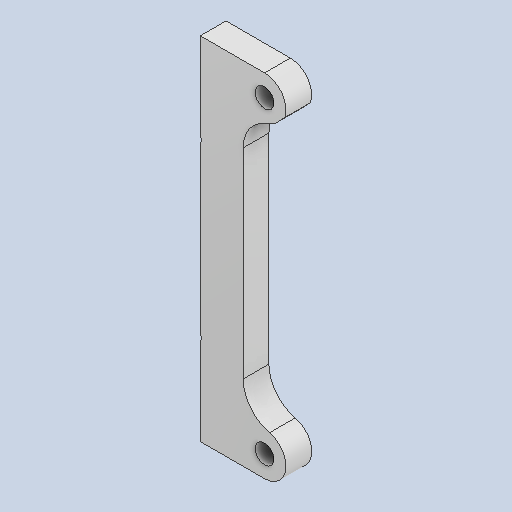
# Autodesk Inventor part: asikubi_asi
Saved by Autodesk Inventor 2025.1 (Build 291241000, 241)
## iProperties
Created: 2024-09-04
Part Number: asikubi_asi
Material: アルミニウム 2014-T4
Document SubType Name: Modeling
Designer: right
Mass: 2.02961 g
Surface Area: 8.92345 cm^2
Volume: 0.724859 cm^3
Density: 2.8 g/cm^3
Appearance: サテン
Author: right
Autodesk Inventor part; units mm, degrees
note: some values were not read from the file. Chosen so that the rebuilt part matches the saved one: edges of "フィレット3".
ref_plane "YZ Plane" through (0, 0, 0) normal (1, 0, 0) x (0, 1, 0)
ref_plane "XZ Plane" through (0, 0, 0) normal (0, 1, 0) x (-1, 0, 0)
ref_plane "XY Plane" through (0, 0, 0) normal (0, 0, 1) x (1, 0, 0)
sketch "スケッチ1" plane through (0, 0, 0) normal (0, 0, 1) x (1, 0, 0)
  line L0 (22.7151, -43.926) -> (22.7151, -4.926) construction
  arc A0 (22.2151, -44.426) -> (22.7151, -43.926) centre (22.2151, -43.926) ccw construction
  line L1 (3.2151, -44.426) -> (22.2151, -44.426) construction
  arc A1 (2.7151, -43.926) -> (3.2151, -44.426) centre (3.2151, -43.926) ccw construction
  line L2 (2.7151, -4.926) -> (2.7151, -43.926) construction
  arc A2 (3.2151, -4.426) -> (2.7151, -4.926) centre (3.2151, -4.926) ccw construction
  line L3 (22.2151, -4.426) -> (3.2151, -4.426) construction
  arc A3 (22.7151, -4.926) -> (22.2151, -4.426) centre (22.2151, -4.926) ccw construction
  line L4 (6.2865, -24.2474) -> (6.2865, -30.6046) construction
  line L5 (6.2865, -30.6046) -> (10.1437, -30.6046) construction
  line L6 (10.1437, -30.6046) -> (10.1437, -24.2474) construction
  line L7 (10.1437, -24.2474) -> (6.2865, -24.2474) construction
  circle A4 centre (12.7151, -31.826) radius 1.1519 construction
  line L8 (19.1437, -24.2474) -> (15.2865, -24.2474) construction
  line L9 (15.2865, -24.2474) -> (15.2865, -30.6046) construction
  line L10 (15.2865, -30.6046) -> (19.1437, -30.6046) construction
  line L11 (19.1437, -30.6046) -> (19.1437, -24.2474) construction
  circle A5 centre (4.7151, -6.426) radius 1.8131 construction
  circle A6 centre (20.7151, -6.426) radius 1.8131 construction
  circle A7 centre (4.7151, -42.426) radius 1.8131 construction
  circle A8 centre (20.7151, -42.426) radius 1.8131 construction
  arc A9 (18.9651, -12.926) -> (6.4651, -12.9153) centre (12.7151, -12.926) ccw construction
  arc A10 (6.4649, -12.9153) -> (6.2151, -12.676) centre (6.2151, -12.926) ccw construction
  line L12 (6.2151, -12.676) -> (4.4651, -12.676) construction
  arc A11 (4.4651, -12.676) -> (4.4651, -13.176) centre (4.4651, -12.926) ccw construction
  line L13 (4.4651, -13.176) -> (6.2151, -13.176) construction
  arc A12 (6.2151, -13.176) -> (6.4651, -12.926) centre (6.2151, -12.926) ccw construction
  arc A13 (6.4651, -12.926) -> (6.9408, -15.3178) centre (12.7151, -12.926) ccw construction
  arc A14 (6.9408, -15.3178) -> (6.6142, -15.1825) centre (6.7099, -15.4134) ccw construction
  line L14 (6.6142, -15.1825) -> (4.9974, -15.8522) construction
  arc A15 (4.9974, -15.8522) -> (5.1888, -16.3141) centre (5.0931, -16.0831) ccw construction
  line L15 (5.1888, -16.3141) -> (6.8055, -15.6444) construction
  arc A16 (6.8055, -15.6444) -> (6.9408, -15.3178) centre (6.7099, -15.4134) ccw construction
  arc A17 (6.9408, -15.3178) -> (8.2957, -17.3454) centre (12.7151, -12.926) ccw construction
  arc A18 (8.2957, -17.3454) -> (7.9421, -17.3454) centre (8.1189, -17.5222) ccw construction
  line L16 (7.9421, -17.3454) -> (6.7047, -18.5829) construction
  arc A19 (6.7047, -18.5829) -> (7.0582, -18.9364) centre (6.8815, -18.7596) ccw construction
  line L17 (7.0582, -18.9364) -> (8.2957, -17.699) construction
  arc A20 (8.2957, -17.699) -> (8.2957, -17.3454) centre (8.1189, -17.5222) ccw construction
  arc A21 (8.2957, -17.3454) -> (10.3233, -18.7003) centre (12.7151, -12.926) ccw construction
  arc A22 (10.3233, -18.7003) -> (9.9967, -18.8356) centre (10.2277, -18.9312) ccw construction
  line L18 (9.9967, -18.8356) -> (9.327, -20.4523) construction
  arc A23 (9.327, -20.4523) -> (9.7889, -20.6437) centre (9.558, -20.548) ccw construction
  line L19 (9.7889, -20.6437) -> (10.4586, -19.0269) construction
  arc A24 (10.4586, -19.0269) -> (10.3233, -18.7003) centre (10.2277, -18.9312) ccw construction
  arc A25 (10.3233, -18.7003) -> (12.7151, -19.176) centre (12.7151, -12.926) ccw construction
  arc A26 (12.7151, -19.176) -> (12.4651, -19.426) centre (12.7151, -19.426) ccw construction
  line L20 (12.4651, -19.426) -> (12.4651, -21.176) construction
  arc A27 (12.4651, -21.176) -> (12.9651, -21.176) centre (12.7151, -21.176) ccw construction
  line L21 (12.9651, -21.176) -> (12.9651, -19.426) construction
  arc A28 (12.9651, -19.426) -> (12.7151, -19.176) centre (12.7151, -19.426) ccw construction
  arc A29 (12.7151, -19.176) -> (15.1069, -18.7003) centre (12.7151, -12.926) ccw construction
  arc A30 (15.1069, -18.7003) -> (14.9716, -19.0269) centre (15.2025, -18.9312) ccw construction
  line L22 (14.9716, -19.0269) -> (15.6413, -20.6437) construction
  arc A31 (15.6413, -20.6437) -> (16.1032, -20.4523) centre (15.8722, -20.548) ccw construction
  line L23 (16.1032, -20.4523) -> (15.4335, -18.8356) construction
  arc A32 (15.4335, -18.8356) -> (15.1069, -18.7003) centre (15.2025, -18.9312) ccw construction
  arc A33 (15.1069, -18.7003) -> (17.1345, -17.3454) centre (12.7151, -12.926) ccw construction
  arc A34 (17.1345, -17.3454) -> (17.1345, -17.699) centre (17.3113, -17.5222) ccw construction
  line L24 (17.1345, -17.699) -> (18.3719, -18.9364) construction
  arc A35 (18.3719, -18.9364) -> (18.7255, -18.5829) centre (18.5487, -18.7596) ccw construction
  line L25 (18.7255, -18.5829) -> (17.4881, -17.3454) construction
  arc A36 (17.4881, -17.3454) -> (17.1345, -17.3454) centre (17.3113, -17.5222) ccw construction
  arc A37 (17.1345, -17.3454) -> (18.4893, -15.3178) centre (12.7151, -12.926) ccw construction
  arc A38 (18.4893, -15.3178) -> (18.6246, -15.6444) centre (18.7203, -15.4134) ccw construction
  line L26 (18.6246, -15.6444) -> (20.2414, -16.3141) construction
  arc A39 (20.2414, -16.3141) -> (20.4328, -15.8522) centre (20.3371, -16.0831) ccw construction
  line L27 (20.4328, -15.8522) -> (18.816, -15.1825) construction
  arc A40 (18.816, -15.1825) -> (18.4893, -15.3178) centre (18.7203, -15.4134) ccw construction
  arc A41 (18.4893, -15.3178) -> (18.9651, -12.926) centre (12.7151, -12.926) ccw construction
  arc A42 (18.9651, -12.926) -> (19.2151, -13.176) centre (19.2151, -12.926) ccw construction
  line L28 (19.2151, -13.176) -> (20.9651, -13.176) construction
  arc A43 (20.9651, -13.176) -> (20.9651, -12.676) centre (20.9651, -12.926) ccw construction
  line L29 (20.9651, -12.676) -> (19.2151, -12.676) construction
  arc A44 (19.2151, -12.676) -> (18.9651, -12.926) centre (19.2151, -12.926) ccw construction
  circle A45 centre (4.7151, -6.426) radius 1.1
  circle A46 centre (4.7151, -42.426) radius 1.1
  circle A47 centre (4.7151, -6.426) radius 2.5
  circle A48 centre (4.7151, -42.426) radius 2.5
  circle A49 centre (12.7151, -12.926) radius 8 construction
  circle A50 centre (12.7151, -12.926) radius 8
  line L30 (12.1437, -22.2474) -> (12.1437, -32.6046)
  line L31 (12.1437, -32.6046) -> (4.2865, -32.6046)
  line L32 (4.2865, -32.6046) -> (4.2865, -22.2474)
  line L33 (4.2865, -22.2474) -> (12.1437, -22.2474)
  line L34 (7.2151, -6.426) -> (7.2151, -42.426)
  line L35 (4.7151, -3.926) -> (-2.7849, -3.926)
  line L36 (-2.7849, -3.926) -> (-2.7849, -44.926)
  line L37 (-2.7849, -44.926) -> (4.7151, -44.926)
  circle A51 centre (-3.7849, -14.426) radius 1.1
  line L38 (7.2151, -24.426) -> (-2.7849, -24.426) construction
  circle A52 centre (-3.7849, -34.426) radius 1.1
  point P0 (0, 0)
  point P1 (7.0743, -7.2531)
  point P2 (-2.7849, -13.9677)
  point P3 (-2.7849, -14.8843)
  point P4 (-2.7849, -33.9677)
  point P5 (-2.7849, -34.8843)
  point P6 (7.2151, -32.6046)
  point P7 (7.2151, -22.2474)
  point P8 (7.2151, -18.7355)
  point P9 (7.2151, -7.1165)
  dimension "d0" = 2.2
  dimension "d1" = 2.2
  dimension "d3" = 5
  dimension "d4" = 5
  dimension "d5" = 2
  dimension "d6" = 10
  dimension "d7" = 2.2
  dimension "d8" = 1
  dimension "d9" = 10
  constraints: 18 end point, 7 centre point, 5 coincident, 4 point on circle, 4 tangent, 2 midpoint, 2 parallel, 1 concentric, 1 perpendicular, 1 symmetric about line, 4 other
  measures "d0" diameter of A45
  measures "d1" diameter of A46
  measures "d3" diameter of A47
  measures "d4" diameter of A48
  measures "d5" distance between parallel lines of L6 L30
  measures "d6" distance between parallel lines of L36 L34
  measures "d7" diameter of A51
  measures "d8" distance from line of L36 A51.centre
  measures "d9" distance from line of L38 A51.centre
extrude "押し出し1" add sketch "スケッチ1" along normal blind 3 contours A47 A50 | L34 A50 A47 | A47 A50 L34 L33 L32 L31 A48 L37 L36 A52 A51 L35 | A48 picked at (5.5204, -8.2788) picked at (7.1889, -6.9354)
fillet "フィレット1" radius 2 4 edges at (7.2151, -22.2474, 1.5) (7.2151, -32.6046, 1.5) (4.2865, -32.6046, 1.5) (4.2865, -22.2474, 1.5)
sketch "スケッチ2" plane through (-2.7849, -33.9677, 0) normal (-1, 0, 0) x (0, 0, 1)
  line L0 (0, 20) -> (3, 20) projected
  line L1 (3, 20) -> (3, 19.0835) projected
  line L2 (3, 0) -> (3, -0.9165) projected
  point P0 (0, 33.9677)
  point P1 (1.5, 19.5417)
  point P2 (1.5, 20)
  point P3 (3, 19.5417)
  point P4 (1.5, -0.4583)
  point P5 (3, -0.4583)
  constraints: 3 midpoint, 2 horizontal alignment, 2 vertical alignment
hole "穴1" at (-2.7849, -14.426, 1.5) at (-2.7849, -34.426, 1.5) direction (1, 0, 0) diameter 1.567 depth 4.3 tip angle 118 thread size "M2x0.4" class "6H" standard "ISO Metric profile"
sketch "スケッチ3" plane through (0, 0, 3) normal (0, 0, 1) x (1, 0, 0)
  circle A0 centre (4.7151, -6.426) radius 1.1 projected
  arc A1 (7.2151, -6.426) -> (4.7151, -3.926) centre (4.7151, -6.426) ccw projected
  circle A2 centre (4.7151, -42.426) radius 1.1 projected
  arc A3 (4.7151, -44.926) -> (7.2151, -42.426) centre (4.7151, -42.426) ccw projected
  circle A4 centre (4.7151, -42.426) radius 2.5
  line L0 (4.7151, -8.926) -> (2.2151, -8.926)
  line L1 (2.2151, -8.926) -> (2.2151, -39.926)
  line L2 (2.2151, -39.926) -> (4.7151, -39.926)
  line L3 (-2.7849, -3.926) -> (-2.7849, -44.926) projected
  arc A5 (5.7508, -22.1743) -> (7.2151, -20.2474) centre (5.2151, -20.2474) ccw projected
  line L4 (7.2151, -20.2474) -> (7.2151, -18.7355) projected
  arc A6 (7.2151, -6.426) -> (4.7151, -3.926) centre (4.7151, -6.426) ccw projected
  line L5 (4.7151, -3.926) -> (-2.7849, -3.926) projected
  line L6 (-2.7849, -3.926) -> (-2.7849, -13.9677) projected
  line L7 (-2.7849, -44.926) -> (4.7151, -44.926) projected
  arc A7 (4.7151, -44.926) -> (7.2151, -42.426) centre (4.7151, -42.426) ccw projected
  line L8 (7.2151, -42.426) -> (7.2151, -34.6046) projected
  arc A8 (7.2151, -34.6046) -> (5.7508, -32.6777) centre (5.2151, -34.6046) ccw projected
  circle A9 centre (4.7151, -42.426) radius 1.1 projected
  circle A10 centre (4.7151, -6.426) radius 1.1 projected
  line L9 (4.2865, -30.7508) -> (4.2865, -24.1012) projected
  arc A11 (5.7508, -22.1743) -> (4.2865, -24.1012) centre (6.2865, -24.1012) ccw projected
  arc A12 (4.2865, -30.7508) -> (5.7508, -32.6777) centre (6.2865, -30.7508) ccw projected
  arc A13 (-2.7849, -14.8843) -> (-2.7849, -13.9677) centre (-3.7849, -14.426) ccw projected
  line L10 (-2.7849, -14.8843) -> (-2.7849, -33.9677) projected
  arc A14 (-2.7849, -34.8843) -> (-2.7849, -33.9677) centre (-3.7849, -34.426) ccw projected
  line L11 (-2.7849, -34.8843) -> (-2.7849, -44.926) projected
  circle A15 centre (4.7151, -6.426) radius 2.5
  arc A16 (7.2151, -7.1165) -> (7.2151, -18.7355) centre (12.7151, -12.926) ccw projected
  line L12 (7.2151, -7.1165) -> (7.2151, -6.426) projected
  point P0 (0, 0)
  point P1 (7.0743, -7.2531)
  point P2 (-2.7849, -14.8843)
  point P3 (-2.7849, -34.8843)
  point P4 (7.0743, -7.2531)
  point P5 (6.0077, -8.5659)
  dimension "d20" = 5
  constraints: 6 end point, 2 coincident, 2 horizontal, 2 perpendicular, 2 point on circle, 1 centre point, 1 tangent, 3 other
  measures "d20" distance between parallel lines of L3 L1
extrude "押し出し2" cut sketch "スケッチ3" against normal through all contours A0 | L12 A16 A15 | A15 A16 L4 A5 A11 L9 A12 A8 L8 A4 L2 L1 L0 | A13 L3 | A14 L3
fillet "フィレット2" radius 4 2 edges at (2.2151, -8.926, 1.5) (2.2151, -39.926, 1.5)
fillet "フィレット3" radius 4 1 edges at (6.0077, -8.5659, 1.5)
